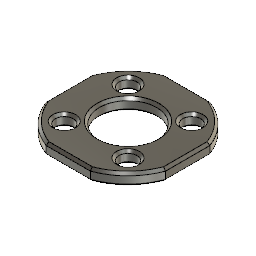
OmniHubSpacer3mm (Autodesk Fusion 360 design; units mm, degrees)
Autodesk Fusion 360 part; units mm, degrees
sketch "Sketch1" plane through (0, 0, 0) normal (0, 0, 1) x (1, 0, 0)
  line L0 (-15, -15) -> (-15, 15)
  line L1 (15, -15) -> (-15, -15)
  line L2 (-6.6408, 2.65) -> (6.6408, 2.65)
  circle A0 centre (-8, -8) radius 2.25
  circle A1 centre (8, 8) radius 2.25
  circle A2 centre (0, 0) radius 16
  circle A3 centre (0, 0) radius 7.15
  line L3 (15, 15) -> (15, -15)
  line L4 (-15, 15) -> (15, 15)
  line L5 (15, 15) -> (-15, -15) construction
  line L6 (-15, 15) -> (15, -15) construction
  circle A4 centre (8, -8) radius 2.25
  circle A5 centre (-8, 8) radius 2.25
  dimension "d2" = 360
  dimension "d3" = 32
  dimension "d4" = 14.3
  dimension "d5" = 2.65
  dimension "d6" = 4.5
  dimension "d7" = 8
  dimension "d8" = 8
  dimension "d9" = 15
  dimension "d10" = 15
  constraint coincident A2.centre A3.centre
  constraint concentric A2 A3
  constraint coincident L2.start A3
  constraint coincident L2.end A3
  constraint horizontal L2
  constraint horizontal L4
  constraint perpendicular L3 L4
  constraint parallel L1 L4
  constraint parallel L0 L3
  constraint coincident A2.centre L6
  constraint coincident A2.centre L5
  measures "d3" diameter of A2
  measures "d4" diameter of A3
  measures "d5" distance of A2.centre L2
  measures "d6" diameter of A5
  measures "d7" horizontal distance of A2.centre A5.centre
  measures "d8" vertical distance of A2.centre A5.centre
  measures "d9" distance of A2.centre L4
  measures "d10" distance of A2.centre L3
extrude "Extrude1" add sketch "Sketch1" along normal blind 3 contours L0 L1 A2 L3 L4
chamfer "Chamfer1" distance 0.6 angle 45 2 faces at (-12.379, -0.144, 0) (-12.379, -0.144, 3)
sketch "Sketch2" plane through (0, 0, 0) normal (1, 0, 0) x (0, 1, 0)
